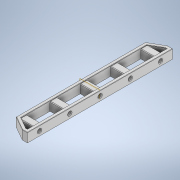
# Autodesk Inventor part: A-00
Saved by Autodesk Inventor 2022 (Build 260153000, 153)
## iProperties
Created: 2021-10-10
Part Number: A-00
Material: Generic
Document SubType Name: Modeling
Designer: kfcs7
Density: 1 g/cm^3
Appearance: Default
Author: kfcs7
Autodesk Inventor part; units mm, degrees
ref_plane "YZ Plane" through (0, 0, 0) normal (1, 0, 0) x (0, 1, 0)
ref_plane "XZ Plane" through (0, 0, 0) normal (0, 1, 0) x (-1, 0, 0)
ref_plane "XY Plane" through (0, 0, 0) normal (0, 0, 1) x (1, 0, 0)
sketch "Sketch2" plane through (0, 0, 0) normal (0, 1, 0) x (-1, 0, 0)
  line L0 (0, 0) -> (31.75, 0)
  line L1 (31.75, 0) -> (31.75, -250)
  line L2 (31.75, -250) -> (0, -250)
  line L3 (0, -250) -> (0, 0)
  dimension "d4" = 31.75
  dimension "d5" = 250
  constraints: 8 end point, 2 parallel, 1 horizontal, 1 perpendicular
  measures "d4" distance of L1.end L2.end
  measures "d5" distance of L0.end L1.end
extrude "Extrusion2" add sketch "Sketch2" along normal blind 15
ref_plane "Work Plane1" through (-31.75, 0, -125) normal (0, 0, 1) x (1, 0, 0)
sketch "Sketch3" plane through (0, 15, 0) normal (0, 1, 0) x (1, 0, 0)
  line L0 (0, 250) -> (-31.75, 250) projected
  line L1 (-31.75, 250) -> (-31.75, 0) projected
  line L2 (-31.75, 0) -> (0, 0) projected
  line L3 (0, 0) -> (0, 250) projected
  line L4 (-31.75, 0) -> (0, 0) projected
  line L5 (0, 0) -> (-31.75, 18.3309)
  line L6 (-31.75, 250) -> (-31.75, 0) projected
  line L7 (0, 0) -> (0, 250) projected
  line L8 (0, 5) -> (-8.6603, 5)
  point P0 (-31.75, 18.3309)
  dimension "d8" = 30
  dimension "d11" = 5
  constraints: 4 end point, 3 point on line, 1 perpendicular
  measures "d8" angle of L2 L5
  measures "d11" distance from line of L4.end L8
extrude "Extrusion3" cut sketch "Sketch3" against normal blind 15 contours L3 L5 L8 | L5 L2 L1
mirror "Mirror1" about plane through (-31.75, 0, -125) normal (0, 0, 1) of "Extrusion3"
shell "Shell1" thickness 5 removed faces 2 at (-10.5833, 15, -89.4436) at (-10.5833, 0, -89.4436)
sketch "Sketch5" plane through (-31.75, 0, -18.3309) normal (-1, 0, 0) x (0, 0, 1)
  line L0 (-213.3383, 15) -> (-213.3383, 0) projected
  line L1 (-213.3383, 0) -> (0, 0) projected
  line L2 (0, 0) -> (0, 15) projected
  line L3 (-213.3383, 15) -> (0, 15) projected
  line L4 (-112.6691, 15) -> (-100.6691, 15)
  line L5 (-100.6691, 15) -> (-100.6691, 0)
  line L6 (-100.6691, 0) -> (-112.6691, 0)
  line L7 (-112.6691, 0) -> (-112.6691, 15)
  line L8 (-112.6691, 15) -> (-100.6691, 0) construction
  line L9 (-100.6691, 15) -> (-112.6691, 0) construction
  line L10 (-213.3383, 15) -> (0, 15) projected
  line L11 (-106.6691, 15) -> (-106.6691, 7.5) construction
  line L12 (0, 0) -> (0, 15) projected
  line L13 (0, 7.5) -> (-106.6691, 7.5) construction
  line L14 (-112.6691, 14) -> (-100.6691, 14)
  point P0 (18.3309, 0)
  point P1 (-112.6691, 0)
  point P2 (-100.6691, 0)
  dimension "d15" = 213.3383
  dimension "d17" = 12
  dimension "d18" = 15
  dimension "d19" = 7.5
  dimension "d20" = 1
  constraints: 18 end point, 3 midpoint, 3 perpendicular, 2 parallel, 2 point on line, 1 horizontal
  measures "d15" distance of L0.start L2.end
  measures "d17" distance of L5.end L6.end
  measures "d18" distance of L4.end L5.end
  measures "d19" distance of L11.start L11.end
  measures "d20" distance between parallel lines of L4 L14
extrude "Extrusion4" add sketch "Sketch5" against normal through all contours L7 L14 L5 L1
sketch "Sketch7" plane through (-31.75, 0, -18.3309) normal (-1, 0, 0) x (0, 0, 1)
  line L0 (-112.6691, 14) -> (-112.6691, 0) projected
  line L1 (-100.6691, 14) -> (-112.6691, 14) projected
  line L2 (-100.6691, 0) -> (-100.6691, 14) projected
  circle A0 centre (-106.6691, 7) radius 2.75
  point P0 (18.3309, 0)
  dimension "d26" = 5.5
  dimension "d27" = 14
  dimension "d28" = 7
  dimension "d29" = 12
  dimension "d30" = 6
  constraints: 1 centre point
  measures "d26" diameter of A0
  measures "d27" distance of L2.start L1.start
  measures "d28" distance from line of L1 A0.centre
  measures "d29" distance of L1.start L0.start
  measures "d30" distance from line of L2 A0.centre
extrude "Extrusion5" cut sketch "Sketch7" against normal through all
chamfer "Chamfer1" distance 3 angle 45 1 edges at (-31.75, 7, -127.75)
chamfer "Chamfer2" distance 1 angle 45 2 edges at (-15.875, 14, -131) (-15.875, 14, -119)
chamfer "Chamfer3" distance 1 angle 45 1 edges at (0, 7, -127.75)
pattern_linear "Rectangular Pattern1" count 5 spacing 50 along (0, 0, 1) of "Extrusion4", "Extrusion5", "Chamfer1", "Chamfer3", "Chamfer2" first direction both ways yes
fillet "Fillet1" radius 0.5 12 edges at (0, 15, -125) (-4.3301, 15, -245) (-20.2051, 15, -238.3346) (-31.75, 15, -125) (-20.2051, 15, -11.6654) (-4.3301, 15, -5) (-17.0353, 15, -234.3912) (-6.1603, 15, -240) (-5, 15, -125) (-26.75, 15, -125) (-17.0353, 15, -15.6088) (-6.1603, 15, -10)
equation "\"d4\" = width"
equation "\"d5\" = length"
equation "\"d6\" = height"
equation "\"d8\" = slam"
equation "\"d11\" = edge_join"
equation "\"d9\" = height"
equation "\"d12\" = wall"
equation "\"d18\" = height"
equation "\"d19\" = 0.5 * height"
equation "\"d28\" = 0.5 * d27"
equation "\"d30\" = 0.5 * d29"
equation "\"width\" = 31.75"
equation "\"length\" = 250"
equation "\"height\" = 15"
equation "\"slam\" = 30deg"
equation "\"edge_join\" = 5"
equation "\"wall\" = 5"
body "Solid2"
